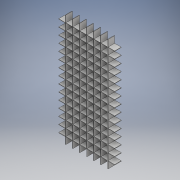
# Autodesk Inventor part: tetris matrix
Saved by Autodesk Inventor 2017 (Build 210142000, 142)
## iProperties
Created: 2019-08-23
Part Number: tetris matrix
Material: Generic
Document SubType Name: Modeling
Designer: EDMU0006
Density: 1 g/cm^3
Appearance: Default
Author: EDMU0006
Autodesk Inventor part; units mm, degrees
ref_plane "YZ Plane" through (0, 0, 0) normal (1, 0, 0) x (0, 1, 0)
ref_plane "XZ Plane" through (0, 0, 0) normal (0, 1, 0) x (-1, 0, 0)
ref_plane "XY Plane" through (0, 0, 0) normal (0, 0, 1) x (1, 0, 0)
sketch "Sketch1" plane through (0, 0, 0) normal (0, 0, 1) x (1, 0, 0)
  line L0 (-159.3068, 381.1292) -> (179.5292, 381.1292)
  line L1 (179.5292, 381.1292) -> (179.5292, -299.0828)
  line L2 (179.5292, -299.0828) -> (-159.3068, -299.0828)
  line L3 (-159.3068, -299.0828) -> (-159.3068, 381.1292)
  point P0 (0, 0)
  dimension "d0" = 338.836
  dimension "d1" = 680.212
  constraints: 8 end point, 2 parallel, 1 horizontal, 1 perpendicular
  measures "d0" distance of L1.end L2.end
  measures "d1" distance of L2.end L0.start
extrude "Extrusion1" add sketch "Sketch1" along normal blind 40.132
sketch "Sketch2" plane through (0, 0, 40.132) normal (0, 0, 1) x (1, 0, 0)
  line L0 (-159.3068, 381.1292) -> (-159.3068, -299.0828) projected
  line L1 (-159.3068, 381.1292) -> (-119.1748, 381.1292)
  line L2 (-119.1748, 381.1292) -> (-119.1748, 340.9972)
  line L3 (-119.1748, 340.9972) -> (-159.3068, 340.9972)
  line L4 (-159.3068, 340.9972) -> (-159.3068, 381.1292)
  line L5 (-159.3068, 338.4572) -> (-119.1748, 338.4572)
  line L6 (-119.1748, 338.4572) -> (-119.1748, 298.3252)
  line L7 (-119.1748, 298.3252) -> (-159.3068, 298.3252)
  line L8 (-159.3068, 298.3252) -> (-159.3068, 338.4572)
  line L9 (-159.3068, 295.7852) -> (-119.1748, 295.7852)
  line L10 (-119.1748, 295.7852) -> (-119.1748, 255.6532)
  line L11 (-119.1748, 255.6532) -> (-159.3068, 255.6532)
  line L12 (-159.3068, 255.6532) -> (-159.3068, 295.7852)
  line L13 (-159.3068, 253.1132) -> (-119.1748, 253.1132)
  line L14 (-119.1748, 253.1132) -> (-119.1748, 212.9812)
  line L15 (-119.1748, 212.9812) -> (-159.3068, 212.9812)
  line L16 (-159.3068, 212.9812) -> (-159.3068, 253.1132)
  line L17 (-159.3068, 210.4412) -> (-119.1748, 210.4412)
  line L18 (-119.1748, 210.4412) -> (-119.1748, 170.3092)
  line L19 (-119.1748, 170.3092) -> (-159.3068, 170.3092)
  line L20 (-159.3068, 170.3092) -> (-159.3068, 210.4412)
  line L21 (-159.3068, 167.7692) -> (-119.1748, 167.7692)
  line L22 (-119.1748, 167.7692) -> (-119.1748, 127.6372)
  line L23 (-119.1748, 127.6372) -> (-159.3068, 127.6372)
  line L24 (-159.3068, 127.6372) -> (-159.3068, 167.7692)
  line L25 (-159.3068, 125.0972) -> (-119.1748, 125.0972)
  line L26 (-119.1748, 125.0972) -> (-119.1748, 84.9652)
  line L27 (-119.1748, 84.9652) -> (-159.3068, 84.9652)
  line L28 (-159.3068, 84.9652) -> (-159.3068, 125.0972)
  line L29 (-159.3068, 82.4252) -> (-119.1748, 82.4252)
  line L30 (-119.1748, 82.4252) -> (-119.1748, 42.2932)
  line L31 (-119.1748, 42.2932) -> (-159.3068, 42.2932)
  line L32 (-159.3068, 42.2932) -> (-159.3068, 82.4252)
  line L33 (-159.3068, 39.7532) -> (-119.1748, 39.7532)
  line L34 (-119.1748, 39.7532) -> (-119.1748, -0.3788)
  line L35 (-119.1748, -0.3788) -> (-159.3068, -0.3788)
  line L36 (-159.3068, -0.3788) -> (-159.3068, 39.7532)
  line L37 (-159.3068, -2.9188) -> (-119.1748, -2.9188)
  line L38 (-119.1748, -2.9188) -> (-119.1748, -43.0508)
  line L39 (-119.1748, -43.0508) -> (-159.3068, -43.0508)
  line L40 (-159.3068, -43.0508) -> (-159.3068, -2.9188)
  line L41 (-159.3068, -45.5908) -> (-119.1748, -45.5908)
  line L42 (-119.1748, -45.5908) -> (-119.1748, -85.7228)
  line L43 (-119.1748, -85.7228) -> (-159.3068, -85.7228)
  line L44 (-159.3068, -85.7228) -> (-159.3068, -45.5908)
  line L45 (-159.3068, -88.2628) -> (-119.1748, -88.2628)
  line L46 (-119.1748, -88.2628) -> (-119.1748, -128.3948)
  line L47 (-119.1748, -128.3948) -> (-159.3068, -128.3948)
  line L48 (-159.3068, -128.3948) -> (-159.3068, -88.2628)
  line L49 (-159.3068, -130.9348) -> (-119.1748, -130.9348)
  line L50 (-119.1748, -130.9348) -> (-119.1748, -171.0668)
  line L51 (-119.1748, -171.0668) -> (-159.3068, -171.0668)
  line L52 (-159.3068, -171.0668) -> (-159.3068, -130.9348)
  line L53 (-159.3068, -173.6068) -> (-119.1748, -173.6068)
  line L54 (-119.1748, -173.6068) -> (-119.1748, -213.7388)
  line L55 (-119.1748, -213.7388) -> (-159.3068, -213.7388)
  line L56 (-159.3068, -213.7388) -> (-159.3068, -173.6068)
  line L57 (-159.3068, -216.2788) -> (-119.1748, -216.2788)
  line L58 (-119.1748, -216.2788) -> (-119.1748, -256.4108)
  line L59 (-119.1748, -256.4108) -> (-159.3068, -256.4108)
  line L60 (-159.3068, -256.4108) -> (-159.3068, -216.2788)
  line L61 (-159.3068, -258.9508) -> (-119.1748, -258.9508)
  line L62 (-119.1748, -258.9508) -> (-119.1748, -299.0828)
  line L63 (-119.1748, -299.0828) -> (-159.3068, -299.0828)
  line L64 (-159.3068, -299.0828) -> (-159.3068, -258.9508)
  line L65 (179.5292, 381.1292) -> (-159.3068, 381.1292) projected
  line L66 (-116.6348, 381.1292) -> (-76.5028, 381.1292)
  line L67 (-76.5028, 381.1292) -> (-76.5028, 340.9972)
  line L68 (-76.5028, 340.9972) -> (-116.6348, 340.9972)
  line L69 (-116.6348, 340.9972) -> (-116.6348, 381.1292)
  line L70 (-73.9628, 381.1292) -> (-33.8308, 381.1292)
  line L71 (-33.8308, 381.1292) -> (-33.8308, 340.9972)
  line L72 (-33.8308, 340.9972) -> (-73.9628, 340.9972)
  line L73 (-73.9628, 340.9972) -> (-73.9628, 381.1292)
  line L74 (-31.2908, 381.1292) -> (8.8412, 381.1292)
  line L75 (8.8412, 381.1292) -> (8.8412, 340.9972)
  line L76 (8.8412, 340.9972) -> (-31.2908, 340.9972)
  line L77 (-31.2908, 340.9972) -> (-31.2908, 381.1292)
  line L78 (11.3812, 381.1292) -> (51.5132, 381.1292)
  line L79 (51.5132, 381.1292) -> (51.5132, 340.9972)
  line L80 (51.5132, 340.9972) -> (11.3812, 340.9972)
  line L81 (11.3812, 340.9972) -> (11.3812, 381.1292)
  line L82 (54.0532, 381.1292) -> (94.1852, 381.1292)
  line L83 (94.1852, 381.1292) -> (94.1852, 340.9972)
  line L84 (94.1852, 340.9972) -> (54.0532, 340.9972)
  line L85 (54.0532, 340.9972) -> (54.0532, 381.1292)
  line L86 (96.7252, 381.1292) -> (136.8572, 381.1292)
  line L87 (136.8572, 381.1292) -> (136.8572, 340.9972)
  line L88 (136.8572, 340.9972) -> (96.7252, 340.9972)
  line L89 (96.7252, 340.9972) -> (96.7252, 381.1292)
  line L90 (139.3972, 381.1292) -> (179.5292, 381.1292)
  line L91 (179.5292, 381.1292) -> (179.5292, 340.9972)
  line L92 (179.5292, 340.9972) -> (139.3972, 340.9972)
  line L93 (139.3972, 340.9972) -> (139.3972, 381.1292)
  line L94 (-116.6348, 338.9652) -> (-76.8843, 338.9652)
  line L95 (-76.8843, 338.9652) -> (-76.8843, 298.8332)
  line L96 (-76.8843, 298.8332) -> (-116.6348, 298.8332)
  line L97 (-116.6348, 298.8332) -> (-116.6348, 338.9652)
  line L98 (-73.9628, 338.9652) -> (-33.8308, 338.9652)
  line L99 (-33.8308, 338.9652) -> (-33.8308, 298.8332)
  line L100 (-33.8308, 298.8332) -> (-73.9628, 298.8332)
  line L101 (-73.9628, 298.8332) -> (-73.9628, 338.9652)
  line L102 (-31.2908, 338.9652) -> (8.8412, 338.9652)
  line L103 (8.8412, 338.9652) -> (8.8412, 298.8332)
  line L104 (8.8412, 298.8332) -> (-31.2908, 298.8332)
  line L105 (-31.2908, 298.8332) -> (-31.2908, 338.9652)
  line L106 (11.3812, 338.9652) -> (51.5132, 338.9652)
  line L107 (51.5132, 338.9652) -> (51.5132, 298.8332)
  line L108 (51.5132, 298.8332) -> (11.3812, 298.8332)
  line L109 (11.3812, 298.8332) -> (11.3812, 338.9652)
  line L110 (54.0532, 338.9652) -> (94.1852, 338.9652)
  line L111 (94.1852, 338.9652) -> (94.1852, 298.8332)
  line L112 (94.1852, 298.8332) -> (54.0532, 298.8332)
  line L113 (54.0532, 298.8332) -> (54.0532, 338.9652)
  line L114 (96.7252, 338.9652) -> (136.8572, 338.9652)
  line L115 (136.8572, 338.9652) -> (136.8572, 298.8332)
  line L116 (136.8572, 298.8332) -> (96.7252, 298.8332)
  line L117 (96.7252, 298.8332) -> (96.7252, 338.9652)
  line L118 (139.3972, 338.9652) -> (179.5292, 338.9652)
  line L119 (179.5292, 338.9652) -> (179.5292, 298.8332)
  line L120 (179.5292, 298.8332) -> (139.3972, 298.8332)
  line L121 (139.3972, 298.8332) -> (139.3972, 338.9652)
  line L122 (-116.6348, 296.2932) -> (-76.8843, 296.2932)
  line L123 (-76.8843, 296.2932) -> (-76.8843, 256.1612)
  line L124 (-76.8843, 256.1612) -> (-116.6348, 256.1612)
  line L125 (-116.6348, 256.1612) -> (-116.6348, 296.2932)
  line L126 (-73.9628, 296.2932) -> (-33.8308, 296.2932)
  line L127 (-33.8308, 296.2932) -> (-33.8308, 256.1612)
  line L128 (-33.8308, 256.1612) -> (-73.9628, 256.1612)
  line L129 (-73.9628, 256.1612) -> (-73.9628, 296.2932)
  line L130 (-31.2908, 296.2932) -> (8.8412, 296.2932)
  line L131 (8.8412, 296.2932) -> (8.8412, 256.1612)
  line L132 (8.8412, 256.1612) -> (-31.2908, 256.1612)
  line L133 (-31.2908, 256.1612) -> (-31.2908, 296.2932)
  line L134 (11.3812, 296.2932) -> (51.5132, 296.2932)
  line L135 (51.5132, 296.2932) -> (51.5132, 256.1612)
  line L136 (51.5132, 256.1612) -> (11.3812, 256.1612)
  line L137 (11.3812, 256.1612) -> (11.3812, 296.2932)
  line L138 (54.0532, 296.2932) -> (94.1852, 296.2932)
  line L139 (94.1852, 296.2932) -> (94.1852, 256.1612)
  line L140 (94.1852, 256.1612) -> (54.0532, 256.1612)
  line L141 (54.0532, 256.1612) -> (54.0532, 296.2932)
  line L142 (96.7252, 296.2932) -> (136.8572, 296.2932)
  line L143 (136.8572, 296.2932) -> (136.8572, 256.1612)
  line L144 (136.8572, 256.1612) -> (96.7252, 256.1612)
  line L145 (96.7252, 256.1612) -> (96.7252, 296.2932)
  line L146 (179.5292, -299.0828) -> (179.5292, 381.1292) projected
  line L147 (139.3972, 296.2932) -> (179.5292, 296.2932)
  line L148 (179.5292, 296.2932) -> (179.5292, 256.1612)
  line L149 (179.5292, 256.1612) -> (139.3972, 256.1612)
  line L150 (139.3972, 256.1612) -> (139.3972, 296.2932)
  line L151 (-116.6348, 253.6212) -> (-76.5028, 253.6212)
  line L152 (-76.5028, 253.6212) -> (-76.5028, 213.4892)
  line L153 (-76.5028, 213.4892) -> (-116.6348, 213.4892)
  line L154 (-116.6348, 213.4892) -> (-116.6348, 253.6212)
  line L155 (-73.9628, 253.6212) -> (-33.8308, 253.6212)
  line L156 (-33.8308, 253.6212) -> (-33.8308, 213.4892)
  line L157 (-33.8308, 213.4892) -> (-73.9628, 213.4892)
  line L158 (-73.9628, 213.4892) -> (-73.9628, 253.6212)
  line L159 (-31.2908, 253.6212) -> (8.8412, 253.6212)
  line L160 (8.8412, 253.6212) -> (8.8412, 213.4892)
  line L161 (8.8412, 213.4892) -> (-31.2908, 213.4892)
  line L162 (-31.2908, 213.4892) -> (-31.2908, 253.6212)
  line L163 (11.3812, 253.6212) -> (51.5132, 253.6212)
  line L164 (51.5132, 253.6212) -> (51.5132, 213.4892)
  line L165 (51.5132, 213.4892) -> (11.3812, 213.4892)
  line L166 (11.3812, 213.4892) -> (11.3812, 253.6212)
  line L167 (54.0532, 253.6212) -> (94.1852, 253.6212)
  line L168 (94.1852, 253.6212) -> (94.1852, 213.4892)
  line L169 (94.1852, 213.4892) -> (54.0532, 213.4892)
  line L170 (54.0532, 213.4892) -> (54.0532, 253.6212)
  line L171 (96.7252, 253.6212) -> (136.8572, 253.6212)
  line L172 (136.8572, 253.6212) -> (136.8572, 213.4892)
  line L173 (136.8572, 213.4892) -> (96.7252, 213.4892)
  line L174 (96.7252, 213.4892) -> (96.7252, 253.6212)
  line L175 (139.3972, 253.6212) -> (179.5292, 253.6212)
  line L176 (179.5292, 253.6212) -> (179.5292, 213.4892)
  line L177 (179.5292, 213.4892) -> (139.3972, 213.4892)
  line L178 (139.3972, 213.4892) -> (139.3972, 253.6212)
  line L179 (-116.6348, 210.9492) -> (-76.5028, 210.9492)
  line L180 (-76.5028, 210.9492) -> (-76.5028, 170.8172)
  line L181 (-76.5028, 170.8172) -> (-116.6348, 170.8172)
  line L182 (-116.6348, 170.8172) -> (-116.6348, 210.9492)
  line L183 (-73.9628, 210.9492) -> (-33.8308, 210.9492)
  line L184 (-33.8308, 210.9492) -> (-33.8308, 170.8172)
  line L185 (-33.8308, 170.8172) -> (-73.9628, 170.8172)
  line L186 (-73.9628, 170.8172) -> (-73.9628, 210.9492)
  line L187 (-31.2908, 210.9492) -> (8.8412, 210.9492)
  line L188 (8.8412, 210.9492) -> (8.8412, 170.8172)
  line L189 (8.8412, 170.8172) -> (-31.2908, 170.8172)
  line L190 (-31.2908, 170.8172) -> (-31.2908, 210.9492)
  line L191 (11.3812, 210.9492) -> (51.5132, 210.9492)
  line L192 (51.5132, 210.9492) -> (51.5132, 170.8172)
  line L193 (51.5132, 170.8172) -> (11.3812, 170.8172)
  line L194 (11.3812, 170.8172) -> (11.3812, 210.9492)
  line L195 (54.0532, 210.9492) -> (94.1852, 210.9492)
  line L196 (94.1852, 210.9492) -> (94.1852, 170.8172)
  line L197 (94.1852, 170.8172) -> (54.0532, 170.8172)
  line L198 (54.0532, 170.8172) -> (54.0532, 210.9492)
  line L199 (96.7252, 210.9492) -> (136.8572, 210.9492)
  line L200 (136.8572, 210.9492) -> (136.8572, 170.8172)
  line L201 (136.8572, 170.8172) -> (96.7252, 170.8172)
  line L202 (96.7252, 170.8172) -> (96.7252, 210.9492)
  line L203 (139.3972, 210.9492) -> (179.5292, 210.9492)
  line L204 (179.5292, 210.9492) -> (179.5292, 170.8172)
  line L205 (179.5292, 170.8172) -> (139.3972, 170.8172)
  line L206 (139.3972, 170.8172) -> (139.3972, 210.9492)
  line L207 (-116.6348, 168.2772) -> (-76.5028, 168.2772)
  line L208 (-76.5028, 168.2772) -> (-76.5028, 128.1452)
  line L209 (-76.5028, 128.1452) -> (-116.6348, 128.1452)
  line L210 (-116.6348, 128.1452) -> (-116.6348, 168.2772)
  line L211 (-73.9628, 168.2772) -> (-33.8308, 168.2772)
  line L212 (-33.8308, 168.2772) -> (-33.8308, 128.1452)
  line L213 (-33.8308, 128.1452) -> (-73.9628, 128.1452)
  line L214 (-73.9628, 128.1452) -> (-73.9628, 168.2772)
  line L215 (-31.2908, 168.2772) -> (8.8412, 168.2772)
  line L216 (8.8412, 168.2772) -> (8.8412, 128.1452)
  line L217 (8.8412, 128.1452) -> (-31.2908, 128.1452)
  line L218 (-31.2908, 128.1452) -> (-31.2908, 168.2772)
  line L219 (11.3812, 168.2772) -> (51.5132, 168.2772)
  line L220 (51.5132, 168.2772) -> (51.5132, 128.1452)
  line L221 (51.5132, 128.1452) -> (11.3812, 128.1452)
  line L222 (11.3812, 128.1452) -> (11.3812, 168.2772)
  line L223 (54.0532, 168.2772) -> (94.1852, 168.2772)
  line L224 (94.1852, 168.2772) -> (94.1852, 128.1452)
  line L225 (94.1852, 128.1452) -> (54.0532, 128.1452)
  line L226 (54.0532, 128.1452) -> (54.0532, 168.2772)
  line L227 (96.7252, 168.2772) -> (136.8572, 168.2772)
  line L228 (136.8572, 168.2772) -> (136.8572, 128.1452)
  line L229 (136.8572, 128.1452) -> (96.7252, 128.1452)
  line L230 (96.7252, 128.1452) -> (96.7252, 168.2772)
  line L231 (139.3972, 168.2772) -> (179.5292, 168.2772)
  line L232 (179.5292, 168.2772) -> (179.5292, 128.1452)
  line L233 (179.5292, 128.1452) -> (139.3972, 128.1452)
  line L234 (139.3972, 128.1452) -> (139.3972, 168.2772)
  line L235 (-116.6348, 125.6052) -> (-76.5028, 125.6052)
  line L236 (-76.5028, 125.6052) -> (-76.5028, 85.4732)
  line L237 (-76.5028, 85.4732) -> (-116.6348, 85.4732)
  line L238 (-116.6348, 85.4732) -> (-116.6348, 125.6052)
  line L239 (-73.9628, 125.6052) -> (-33.8308, 125.6052)
  line L240 (-33.8308, 125.6052) -> (-33.8308, 85.4732)
  line L241 (-33.8308, 85.4732) -> (-73.9628, 85.4732)
  line L242 (-73.9628, 85.4732) -> (-73.9628, 125.6052)
  line L243 (-31.2908, 125.6052) -> (8.8412, 125.6052)
  line L244 (8.8412, 125.6052) -> (8.8412, 85.4732)
  line L245 (8.8412, 85.4732) -> (-31.2908, 85.4732)
  line L246 (-31.2908, 85.4732) -> (-31.2908, 125.6052)
  line L247 (11.3812, 125.6052) -> (51.5132, 125.6052)
  line L248 (51.5132, 125.6052) -> (51.5132, 85.4732)
  line L249 (51.5132, 85.4732) -> (11.3812, 85.4732)
  line L250 (11.3812, 85.4732) -> (11.3812, 125.6052)
  line L251 (54.0532, 125.6052) -> (94.1852, 125.6052)
  line L252 (94.1852, 125.6052) -> (94.1852, 85.4732)
  line L253 (94.1852, 85.4732) -> (54.0532, 85.4732)
  line L254 (54.0532, 85.4732) -> (54.0532, 125.6052)
  line L255 (96.7252, 125.6052) -> (136.8572, 125.6052)
  line L256 (136.8572, 125.6052) -> (136.8572, 85.4732)
  line L257 (136.8572, 85.4732) -> (96.7252, 85.4732)
  line L258 (96.7252, 85.4732) -> (96.7252, 125.6052)
  line L259 (139.3972, 125.6052) -> (179.5292, 125.6052)
  line L260 (179.5292, 125.6052) -> (179.5292, 85.4732)
  line L261 (179.5292, 85.4732) -> (139.3972, 85.4732)
  line L262 (139.3972, 85.4732) -> (139.3972, 125.6052)
  line L263 (-116.6348, 82.9332) -> (-76.5028, 82.9332)
  line L264 (-76.5028, 82.9332) -> (-76.5028, 42.8012)
  line L265 (-76.5028, 42.8012) -> (-116.6348, 42.8012)
  line L266 (-116.6348, 42.8012) -> (-116.6348, 82.9332)
  line L267 (-73.9628, 82.9332) -> (-33.8308, 82.9332)
  line L268 (-33.8308, 82.9332) -> (-33.8308, 42.8012)
  line L269 (-33.8308, 42.8012) -> (-73.9628, 42.8012)
  line L270 (-73.9628, 42.8012) -> (-73.9628, 82.9332)
  line L271 (-31.2908, 82.9332) -> (8.8412, 82.9332)
  line L272 (8.8412, 82.9332) -> (8.8412, 42.8012)
  line L273 (8.8412, 42.8012) -> (-31.2908, 42.8012)
  line L274 (-31.2908, 42.8012) -> (-31.2908, 82.9332)
  line L275 (11.3812, 82.9332) -> (51.5132, 82.9332)
  line L276 (51.5132, 82.9332) -> (51.5132, 42.8012)
  line L277 (51.5132, 42.8012) -> (11.3812, 42.8012)
  line L278 (11.3812, 42.8012) -> (11.3812, 82.9332)
  line L279 (54.0532, 82.9332) -> (94.1852, 82.9332)
  line L280 (94.1852, 82.9332) -> (94.1852, 42.8012)
  line L281 (94.1852, 42.8012) -> (54.0532, 42.8012)
  line L282 (54.0532, 42.8012) -> (54.0532, 82.9332)
  line L283 (96.7252, 82.9332) -> (136.8572, 82.9332)
  line L284 (136.8572, 82.9332) -> (136.8572, 42.8012)
  line L285 (136.8572, 42.8012) -> (96.7252, 42.8012)
  line L286 (96.7252, 42.8012) -> (96.7252, 82.9332)
  line L287 (139.3972, 82.9332) -> (179.5292, 82.9332)
  line L288 (179.5292, 82.9332) -> (179.5292, 42.8012)
  line L289 (179.5292, 42.8012) -> (139.3972, 42.8012)
  line L290 (139.3972, 42.8012) -> (139.3972, 82.9332)
  line L291 (-116.6348, 40.2612) -> (-76.5028, 40.2612)
  line L292 (-76.5028, 40.2612) -> (-76.5028, 0.1292)
  line L293 (-76.5028, 0.1292) -> (-116.6348, 0.1292)
  line L294 (-116.6348, 0.1292) -> (-116.6348, 40.2612)
  line L295 (-73.9628, 40.2612) -> (-33.8308, 40.2612)
  line L296 (-33.8308, 40.2612) -> (-33.8308, 0.1292)
  line L297 (-33.8308, 0.1292) -> (-73.9628, 0.1292)
  line L298 (-73.9628, 0.1292) -> (-73.9628, 40.2612)
  line L299 (-31.2908, 40.2612) -> (8.8412, 40.2612)
  line L300 (8.8412, 40.2612) -> (8.8412, 0.1292)
  line L301 (8.8412, 0.1292) -> (-31.2908, 0.1292)
  line L302 (-31.2908, 0.1292) -> (-31.2908, 40.2612)
  line L303 (11.3812, 40.2612) -> (51.5132, 40.2612)
  line L304 (51.5132, 40.2612) -> (51.5132, 0.1292)
  line L305 (51.5132, 0.1292) -> (11.3812, 0.1292)
  line L306 (11.3812, 0.1292) -> (11.3812, 40.2612)
  line L307 (54.0532, 40.2612) -> (94.1852, 40.2612)
  line L308 (94.1852, 40.2612) -> (94.1852, 0.1292)
  line L309 (94.1852, 0.1292) -> (54.0532, 0.1292)
  line L310 (54.0532, 0.1292) -> (54.0532, 40.2612)
  line L311 (96.7252, 40.2612) -> (136.8572, 40.2612)
  line L312 (136.8572, 40.2612) -> (136.8572, 0.1292)
  line L313 (136.8572, 0.1292) -> (96.7252, 0.1292)
  line L314 (96.7252, 0.1292) -> (96.7252, 40.2612)
  line L315 (139.3972, 40.2612) -> (179.5292, 40.2612)
  line L316 (179.5292, 40.2612) -> (179.5292, 0.1292)
  line L317 (179.5292, 0.1292) -> (139.3972, 0.1292)
  line L318 (139.3972, 0.1292) -> (139.3972, 40.2612)
  line L319 (-116.6348, -2.4108) -> (-76.5028, -2.4108)
  line L320 (-76.5028, -2.4108) -> (-76.5028, -42.5428)
  line L321 (-76.5028, -42.5428) -> (-116.6348, -42.5428)
  line L322 (-116.6348, -42.5428) -> (-116.6348, -2.4108)
  line L323 (-73.9628, -2.4108) -> (-33.8308, -2.4108)
  line L324 (-33.8308, -2.4108) -> (-33.8308, -42.5428)
  line L325 (-33.8308, -42.5428) -> (-73.9628, -42.5428)
  line L326 (-73.9628, -42.5428) -> (-73.9628, -2.4108)
  line L327 (-31.2908, -2.4108) -> (8.8412, -2.4108)
  line L328 (8.8412, -2.4108) -> (8.8412, -42.5428)
  line L329 (8.8412, -42.5428) -> (-31.2908, -42.5428)
  line L330 (-31.2908, -42.5428) -> (-31.2908, -2.4108)
  line L331 (11.3812, -2.4108) -> (51.5132, -2.4108)
  line L332 (51.5132, -2.4108) -> (51.5132, -42.5428)
  line L333 (51.5132, -42.5428) -> (11.3812, -42.5428)
  line L334 (11.3812, -42.5428) -> (11.3812, -2.4108)
  line L335 (54.0532, -2.4108) -> (94.1852, -2.4108)
  line L336 (94.1852, -2.4108) -> (94.1852, -42.5428)
  line L337 (94.1852, -42.5428) -> (54.0532, -42.5428)
  line L338 (54.0532, -42.5428) -> (54.0532, -2.4108)
  line L339 (96.7252, -2.4108) -> (136.8572, -2.4108)
  line L340 (136.8572, -2.4108) -> (136.8572, -42.5428)
  line L341 (136.8572, -42.5428) -> (96.7252, -42.5428)
  line L342 (96.7252, -42.5428) -> (96.7252, -2.4108)
  line L343 (139.3972, -2.4108) -> (179.5292, -2.4108)
  line L344 (179.5292, -2.4108) -> (179.5292, -42.5428)
  line L345 (179.5292, -42.5428) -> (139.3972, -42.5428)
  line L346 (139.3972, -42.5428) -> (139.3972, -2.4108)
  line L347 (-116.6348, -45.5908) -> (-76.5028, -45.5908)
  line L348 (-76.5028, -45.5908) -> (-76.5028, -85.7228)
  line L349 (-76.5028, -85.7228) -> (-116.6348, -85.7228)
  line L350 (-116.6348, -85.7228) -> (-116.6348, -45.5908)
  line L351 (-73.9628, -45.5908) -> (-33.8308, -45.5908)
  line L352 (-33.8308, -45.5908) -> (-33.8308, -85.7228)
  line L353 (-33.8308, -85.7228) -> (-73.9628, -85.7228)
  line L354 (-73.9628, -85.7228) -> (-73.9628, -45.5908)
  line L355 (-31.2908, -45.5908) -> (8.8412, -45.5908)
  line L356 (8.8412, -45.5908) -> (8.8412, -85.7228)
  line L357 (8.8412, -85.7228) -> (-31.2908, -85.7228)
  line L358 (-31.2908, -85.7228) -> (-31.2908, -45.5908)
  line L359 (11.3812, -45.5908) -> (51.5132, -45.5908)
  line L360 (51.5132, -45.5908) -> (51.5132, -85.7228)
  line L361 (51.5132, -85.7228) -> (11.3812, -85.7228)
  line L362 (11.3812, -85.7228) -> (11.3812, -45.5908)
  line L363 (54.0532, -45.5908) -> (94.1852, -45.5908)
  line L364 (94.1852, -45.5908) -> (94.1852, -85.7228)
  line L365 (94.1852, -85.7228) -> (54.0532, -85.7228)
  line L366 (54.0532, -85.7228) -> (54.0532, -45.5908)
  line L367 (96.7252, -45.5908) -> (136.8572, -45.5908)
  line L368 (136.8572, -45.5908) -> (136.8572, -85.7228)
  line L369 (136.8572, -85.7228) -> (96.7252, -85.7228)
  line L370 (96.7252, -85.7228) -> (96.7252, -45.5908)
  line L371 (139.3972, -45.5908) -> (179.5292, -45.5908)
  line L372 (179.5292, -45.5908) -> (179.5292, -85.7228)
  line L373 (179.5292, -85.7228) -> (139.3972, -85.7228)
  line L374 (139.3972, -85.7228) -> (139.3972, -45.5908)
  line L375 (-116.6348, -88.2628) -> (-76.5028, -88.2628)
  line L376 (-76.5028, -88.2628) -> (-76.5028, -128.3948)
  line L377 (-76.5028, -128.3948) -> (-116.6348, -128.3948)
  line L378 (-116.6348, -128.3948) -> (-116.6348, -88.2628)
  line L379 (-116.6348, -130.9348) -> (-76.5028, -130.9348)
  line L380 (-76.5028, -130.9348) -> (-76.5028, -171.0668)
  line L381 (-76.5028, -171.0668) -> (-116.6348, -171.0668)
  line L382 (-116.6348, -171.0668) -> (-116.6348, -130.9348)
  line L383 (-116.6348, -173.6068) -> (-76.5028, -173.6068)
  line L384 (-76.5028, -173.6068) -> (-76.5028, -213.7388)
  line L385 (-76.5028, -213.7388) -> (-116.6348, -213.7388)
  line L386 (-116.6348, -213.7388) -> (-116.6348, -173.6068)
  line L387 (-116.6348, -216.2788) -> (-76.5028, -216.2788)
  line L388 (-76.5028, -216.2788) -> (-76.5028, -256.4108)
  line L389 (-76.5028, -256.4108) -> (-116.6348, -256.4108)
  line L390 (-116.6348, -256.4108) -> (-116.6348, -216.2788)
  line L391 (-116.6348, -258.9508) -> (-76.5028, -258.9508)
  line L392 (-76.5028, -258.9508) -> (-76.5028, -299.0828)
  line L393 (-76.5028, -299.0828) -> (-116.6348, -299.0828)
  line L394 (-116.6348, -299.0828) -> (-116.6348, -258.9508)
  line L395 (-73.9628, -88.2628) -> (-33.8308, -88.2628)
  line L396 (-33.8308, -88.2628) -> (-33.8308, -128.3948)
  line L397 (-33.8308, -128.3948) -> (-73.9628, -128.3948)
  line L398 (-73.9628, -128.3948) -> (-73.9628, -88.2628)
  line L399 (-73.9628, -130.9348) -> (-33.8308, -130.9348)
  line L400 (-33.8308, -130.9348) -> (-33.8308, -171.0668)
  line L401 (-33.8308, -171.0668) -> (-73.9628, -171.0668)
  line L402 (-73.9628, -171.0668) -> (-73.9628, -130.9348)
  line L403 (-73.9628, -173.6068) -> (-33.8308, -173.6068)
  line L404 (-33.8308, -173.6068) -> (-33.8308, -213.7388)
  line L405 (-33.8308, -213.7388) -> (-73.9628, -213.7388)
  line L406 (-73.9628, -213.7388) -> (-73.9628, -173.6068)
  line L407 (-73.9628, -216.2788) -> (-33.8308, -216.2788)
  line L408 (-33.8308, -216.2788) -> (-33.8308, -256.4108)
  line L409 (-33.8308, -256.4108) -> (-73.9628, -256.4108)
  line L410 (-73.9628, -256.4108) -> (-73.9628, -216.2788)
  line L411 (-159.3068, -299.0828) -> (179.5292, -299.0828) projected
  line L412 (-73.9628, -258.9508) -> (-33.8308, -258.9508)
  line L413 (-33.8308, -258.9508) -> (-33.8308, -299.0828)
  line L414 (-33.8308, -299.0828) -> (-73.9628, -299.0828)
  line L415 (-73.9628, -299.0828) -> (-73.9628, -258.9508)
  line L416 (-31.2908, -87.7548) -> (8.8412, -87.7548)
  line L417 (8.8412, -87.7548) -> (8.8412, -127.8868)
  line L418 (8.8412, -127.8868) -> (-31.2908, -127.8868)
  line L419 (-31.2908, -127.8868) -> (-31.2908, -87.7548)
  line L420 (-31.2908, -130.4268) -> (8.8412, -130.4268)
  line L421 (8.8412, -130.4268) -> (8.8412, -170.5588)
  line L422 (8.8412, -170.5588) -> (-31.2908, -170.5588)
  line L423 (-31.2908, -170.5588) -> (-31.2908, -130.4268)
  line L424 (-31.2908, -173.0988) -> (8.8412, -173.0988)
  line L425 (8.8412, -173.0988) -> (8.8412, -213.2308)
  line L426 (8.8412, -213.2308) -> (-31.2908, -213.2308)
  line L427 (-31.2908, -213.2308) -> (-31.2908, -173.0988)
  line L428 (-31.2908, -215.7708) -> (8.8412, -215.7708)
  line L429 (8.8412, -215.7708) -> (8.8412, -255.9028)
  line L430 (8.8412, -255.9028) -> (-31.2908, -255.9028)
  line L431 (-31.2908, -255.9028) -> (-31.2908, -215.7708)
  line L432 (-31.2908, -258.9508) -> (10.1112, -258.9508)
  line L433 (10.1112, -258.9508) -> (10.1112, -299.0828)
  line L434 (10.1112, -299.0828) -> (-31.2908, -299.0828)
  line L435 (-31.2908, -299.0828) -> (-31.2908, -258.9508)
  line L436 (11.3812, -87.7548) -> (51.5132, -87.7548)
  line L437 (51.5132, -87.7548) -> (51.5132, -127.8868)
  line L438 (51.5132, -127.8868) -> (11.3812, -127.8868)
  line L439 (11.3812, -127.8868) -> (11.3812, -87.7548)
  line L440 (54.0532, -87.7548) -> (94.1852, -87.7548)
  line L441 (94.1852, -87.7548) -> (94.1852, -127.8868)
  line L442 (94.1852, -127.8868) -> (54.0532, -127.8868)
  line L443 (54.0532, -127.8868) -> (54.0532, -87.7548)
  line L444 (96.7252, -87.7548) -> (136.8572, -87.7548)
  line L445 (136.8572, -87.7548) -> (136.8572, -127.8868)
  line L446 (136.8572, -127.8868) -> (96.7252, -127.8868)
  line L447 (96.7252, -127.8868) -> (96.7252, -87.7548)
  line L448 (139.3972, -87.7548) -> (179.5292, -87.7548)
  line L449 (179.5292, -87.7548) -> (179.5292, -127.8868)
  line L450 (179.5292, -127.8868) -> (139.3972, -127.8868)
  line L451 (139.3972, -127.8868) -> (139.3972, -87.7548)
  line L452 (11.3812, -130.9348) -> (51.5132, -130.9348)
  line L453 (51.5132, -130.9348) -> (51.5132, -170.5588)
  line L454 (51.5132, -170.5588) -> (11.3812, -170.5588)
  line L455 (11.3812, -170.5588) -> (11.3812, -130.9348)
  line L456 (11.3812, -173.6068) -> (51.5132, -173.6068)
  line L457 (51.5132, -173.6068) -> (51.5132, -213.2308)
  line L458 (51.5132, -213.2308) -> (11.3812, -213.2308)
  line L459 (11.3812, -213.2308) -> (11.3812, -173.6068)
  line L460 (11.3812, -216.2788) -> (51.5132, -216.2788)
  line L461 (51.5132, -216.2788) -> (51.5132, -255.9028)
  line L462 (51.5132, -255.9028) -> (11.3812, -255.9028)
  line L463 (11.3812, -255.9028) -> (11.3812, -216.2788)
  line L464 (11.3812, -258.9508) -> (51.5132, -258.9508)
  line L465 (51.5132, -258.9508) -> (51.5132, -299.0828)
  line L466 (51.5132, -299.0828) -> (11.3812, -299.0828)
  line L467 (11.3812, -299.0828) -> (11.3812, -258.9508)
  line L468 (54.0532, -130.9348) -> (94.1852, -130.9348)
  line L469 (94.1852, -130.9348) -> (94.1852, -170.5588)
  line L470 (94.1852, -170.5588) -> (54.0532, -170.5588)
  line L471 (54.0532, -170.5588) -> (54.0532, -130.9348)
  line L472 (54.0532, -173.6068) -> (94.1852, -173.6068)
  line L473 (94.1852, -173.6068) -> (94.1852, -213.2308)
  line L474 (94.1852, -213.2308) -> (54.0532, -213.2308)
  line L475 (54.0532, -213.2308) -> (54.0532, -173.6068)
  line L476 (54.0532, -216.2788) -> (94.1852, -216.2788)
  line L477 (94.1852, -216.2788) -> (94.1852, -255.9028)
  line L478 (94.1852, -255.9028) -> (54.0532, -255.9028)
  line L479 (54.0532, -255.9028) -> (54.0532, -216.2788)
  line L480 (96.7252, -130.9348) -> (136.8572, -130.9348)
  line L481 (136.8572, -130.9348) -> (136.8572, -170.5588)
  line L482 (136.8572, -170.5588) -> (96.7252, -170.5588)
  line L483 (96.7252, -170.5588) -> (96.7252, -130.9348)
  line L484 (139.3972, -130.9348) -> (179.5292, -130.9348)
  line L485 (179.5292, -130.9348) -> (179.5292, -170.5588)
  line L486 (179.5292, -170.5588) -> (139.3972, -170.5588)
  line L487 (139.3972, -170.5588) -> (139.3972, -130.9348)
  line L488 (96.7252, -173.6068) -> (136.8572, -173.6068)
  line L489 (136.8572, -173.6068) -> (136.8572, -213.2308)
  line L490 (136.8572, -213.2308) -> (96.7252, -213.2308)
  line L491 (96.7252, -213.2308) -> (96.7252, -173.6068)
  line L492 (139.3972, -173.6068) -> (179.5292, -173.6068)
  line L493 (179.5292, -173.6068) -> (179.5292, -213.2308)
  line L494 (179.5292, -213.2308) -> (139.3972, -213.2308)
  line L495 (139.3972, -213.2308) -> (139.3972, -173.6068)
  line L496 (96.7252, -216.2788) -> (136.8572, -216.2788)
  line L497 (136.8572, -216.2788) -> (136.8572, -255.9028)
  line L498 (136.8572, -255.9028) -> (96.7252, -255.9028)
  line L499 (96.7252, -255.9028) -> (96.7252, -216.2788)
  line L500 (139.3972, -216.2788) -> (179.5292, -216.2788)
  line L501 (179.5292, -216.2788) -> (179.5292, -255.9028)
  line L502 (179.5292, -255.9028) -> (139.3972, -255.9028)
  line L503 (139.3972, -255.9028) -> (139.3972, -216.2788)
  line L504 (54.0532, -258.9508) -> (94.1852, -258.9508)
  line L505 (94.1852, -258.9508) -> (94.1852, -299.0828)
  line L506 (94.1852, -299.0828) -> (54.0532, -299.0828)
  line L507 (54.0532, -299.0828) -> (54.0532, -258.9508)
  line L508 (96.7252, -258.9508) -> (136.8572, -258.9508)
  line L509 (136.8572, -258.9508) -> (136.8572, -299.0828)
  line L510 (136.8572, -299.0828) -> (96.7252, -299.0828)
  line L511 (96.7252, -299.0828) -> (96.7252, -258.9508)
  line L512 (139.3972, -258.9508) -> (179.5292, -258.9508)
  line L513 (179.5292, -258.9508) -> (179.5292, -299.0828)
  line L514 (179.5292, -299.0828) -> (139.3972, -299.0828)
  line L515 (139.3972, -299.0828) -> (139.3972, -258.9508)
  point P0 (0, 0)
  dimension "d6" = 40.132
  dimension "d11" = 2.54
  dimension "d13" = 2.54
  dimension "d17" = 2.54
  dimension "d22" = 2.54
  dimension "d25" = 2.54
  dimension "d28" = 2.54
  dimension "d30" = 2.54
  dimension "d32" = 2.54
  dimension "d34" = 2.54
  dimension "d38" = 2.54
  dimension "d39" = 2.54
  dimension "d40" = 2.54
  dimension "d44" = 2.54
  dimension "d45" = 2.54
  dimension "d46" = 2.54
  dimension "d53" = 2.54
  dimension "d54" = 2.54
  dimension "d55" = 2.54
  dimension "d56" = 2.54
  dimension "d57" = 2.54
  dimension "d58" = 2.54
  dimension "d60" = 2.54
  dimension "d78" = 40.132
  dimension "d79" = 40.132
  dimension "d80" = 40.132
  dimension "d82" = 40.132
  dimension "d83" = 40.132
  dimension "d84" = 40.132
  dimension "d85" = 40.132
  dimension "d86" = 40.132
  dimension "d87" = 40.132
  dimension "d88" = 40.132
  dimension "d89" = 40.132
  dimension "d90" = 40.132
  dimension "d91" = 40.132
  dimension "d92" = 40.132
  dimension "d93" = 40.132
  dimension "d94" = 40.132
  dimension "d95" = 40.132
  dimension "d96" = 40.132
  dimension "d97" = 40.132
  constraints: 1024 end point, 288 point on line, 256 parallel, 128 horizontal, 128 perpendicular, 1 midpoint, 39 other
  measures "d6" distance of L1.start L1.end
  measures "d11" distance between parallel lines of L5 L3
  measures "d13" distance between parallel lines of L9 L7
  measures "d17" distance between parallel lines of L13 L11
  measures "d22" distance between parallel lines of L17 L15
  measures "d25" distance between parallel lines of L21 L19
  measures "d28" distance between parallel lines of L25 L23
  measures "d30" distance between parallel lines of L29 L27
  measures "d32" distance between parallel lines of L33 L31
  measures "d34" distance between parallel lines of L37 L35
  measures "d38" distance between parallel lines of L41 L39
  measures "d39" distance between parallel lines of L43 L45
  measures "d40" distance between parallel lines of L47 L49
  measures "d44" distance between parallel lines of L53 L51
  measures "d45" distance between parallel lines of L55 L57
  measures "d46" distance between parallel lines of L61 L59
  measures "d53" distance between parallel lines of L2 L69
  measures "d54" distance between parallel lines of L67 L73
  measures "d55" distance between parallel lines of L77 L71
  measures "d56" distance between parallel lines of L81 L75
  measures "d57" distance between parallel lines of L85 L79
  measures "d58" distance between parallel lines of L83 L89
  measures "d60" distance between parallel lines of L93 L87
  measures "d78" distance of L414.end L412.start
  measures "d79" distance of L434.end L432.start
  measures "d80" distance of L466.end L464.start
  measures "d82" distance of L1.end L2.end
  measures "d83" distance of L5.end L6.end
  measures "d84" distance of L9.end L10.end
  measures "d85" distance of L13.end L14.end
  measures "d86" distance of L17.end L18.end
  measures "d87" distance of L21.end L22.end
  measures "d88" distance of L25.end L26.end
  measures "d89" distance of L29.end L30.end
  measures "d90" distance of L33.end L34.end
  measures "d91" distance of L37.end L38.end
  measures "d92" distance of L41.end L42.end
  measures "d93" distance of L45.end L46.end
  measures "d94" distance of L49.end L50.end
  measures "d95" distance of L53.end L54.end
  measures "d96" distance of L57.end L58.end
  measures "d97" distance of L61.end L62.end
extrude "Extrusion2" cut sketch "Sketch2" against normal blind 127 contours L1 L2 L3 L0 | L5 L6 L7 L0 | L65 L67 L68 L69 | L9 L10 L11 L0 | L65 L71 L72 L73 | L13 L14 L15 L0 | L65 L75 L76 L77 | L17 L18 L19 L0 | L65 L79 L80 L81 | L21 L22 L23 L0 | L65 L83 L84 L85 | L25 L26 L27 L0 | L65 L87 L88 L89 | L29 L30 L31 L0 | L65 L91 L92 L93 | L33 L34 L35 L0 | L119 L120 L121 L118 | L37 L38 L39 L0 | L146 L149 L150 L147 | L41 L42 L43 L0 | L146 L177 L178 L175 | L45 L46 L47 L0 | L146 L205 L206 L203 | L49 L50 L51 L0 | L146 L233 L234 L231 | L53 L54 L55 L0 | L146 L261 L262 L259 | L57 L58 L59 L0 | L146 L289 L290 L287 | L61 L62 L63 L0 | L146 L317 L318 L315 | L394 L391 L392 L393 | L146 L345 L346 L343 | L415 L412 L413 L411 | L146 L373 L374 L371 | L435 L432 L433 L411 | L146 L450 L451 L448 | L467 L464 L465 L411 | L146 L486 L487 L484 | L507 L504 L505 L411 | L146 L494 L495 L492 | L511 L508 L509 L411 | L146 L502 L503 L500 | L515 L512 L146 L411 | L94 L95 L96 L97 | L98 L99 L100 L101 | L102 L103 L104 L105 | L106 L107 L108 L109 | L110 L111 L112 L113 | L114 L115 L116 L117 | L122 L123 L124 L125 | L126 L127 L128 L129 | L130 L131 L132 L133 | L134 L135 L136 L137 | L138 L139 L140 L141 | L142 L143 L144 L145 | L151 L152 L153 L154 | L155 L156 L157 L158 | L159 L160 L161 L162 | L163 L164 L165 L166 | L167 L168 L169 L170 | L171 L172 L173 L174 | L179 L180 L181 L182 | L183 L184 L185 L186 | L187 L188 L189 L190 | L191 L192 L193 L194 | L195 L196 L197 L198 | L199 L200 L201 L202 | L207 L208 L209 L210 | L211 L212 L213 L214 | L215 L216 L217 L218 | L219 L220 L221 L222 | L223 L224 L225 L226 | L227 L228 L229 L230 | L235 L236 L237 L238 | L239 L240 L241 L242 | L243 L244 L245 L246 | L247 L248 L249 L250 | L251 L252 L253 L254 | L255 L256 L257 L258 | L263 L264 L265 L266 | L267 L268 L269 L270 | L271 L272 L273 L274 | L275 L276 L277 L278 | L279 L280 L281 L282 | L283 L284 L285 L286 | L291 L292 L293 L294 | L295 L296 L297 L298 | L299 L300 L301 L302 | L303 L304 L305 L306 | L307 L308 L309 L310 | L311 L312 L313 L314 | L319 L320 L321 L322 | L323 L324 L325 L326 | L327 L328 L329 L330 | L331 L332 L333 L334 | L335 L336 L337 L338 | L339 L340 L341 L342 | L347 L348 L349 L350 | L351 L352 L353 L354 | L355 L356 L357 L358 | L359 L360 L361 L362 | L363 L364 L365 L366 | L367 L368 L369 L370 | L375 L376 L377 L378 | L379 L380 L381 L382 | L383 L384 L385 L386 | L387 L388 L389 L390 | L395 L396 L397 L398 | L399 L400 L401 L402 | L403 L404 L405 L406 | L407 L408 L409 L410 | L416 L417 L418 L419 | L420 L421 L422 L423 | L424 L425 L426 L427 | L428 L429 L430 L431 | L436 L437 L438 L439 | L440 L441 L442 L443 | L444 L445 L446 L447 | L452 L453 L454 L455 | L456 L457 L458 L459 | L460 L461 L462 L463 | L468 L469 L470 L471 | L472 L473 L474 L475 | L476 L477 L478 L479 | L480 L481 L482 L483 | L488 L489 L490 L491 | L496 L497 L498 L499
body "Solid1"
